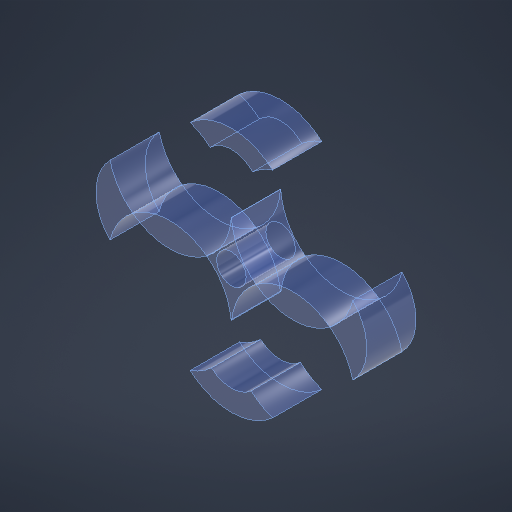
# Autodesk Inventor part: Peça2
Saved by Autodesk Inventor 2026.1 (Build 301233000, 233)
## iProperties
Created: 2025-10-22
Part Number: Peça2
Material: Água
Document SubType Name: Modeling
Designer: Pc
Density: 0.9983 g/cm^3
Appearance: Azul tropical
Author: Pc
Autodesk Inventor part; units mm, degrees
ref_plane "YZ Plane" through (0, 0, 0) normal (1, 0, 0) x (0, 1, 0)
ref_plane "XZ Plane" through (0, 0, 0) normal (0, 1, 0) x (-1, 0, 0)
ref_plane "XY Plane" through (0, 0, 0) normal (0, 0, 1) x (1, 0, 0)
sketch "Esboço1" plane through (0, 0, 0) normal (0, 0, 1) x (1, 0, 0)
  line L0 (30.3854, 49.745) -> (30.3854, 49.745)
  line L1 (42.8854, 37.245) -> (42.8854, 12.245)
  line L2 (30.3854, -0.255) -> (30.3854, -0.255)
  line L3 (17.8854, 12.245) -> (17.8854, 37.245)
  circle A0 centre (30.3854, 25) radius 3
  circle A1 centre (30.3854, 40) radius 6
  circle A2 centre (30.3854, 10) radius 6
  line L4 (47.8854, 34.745) -> (42.8854, 34.745)
  line L5 (42.8854, 34.745) -> (42.8854, 14.745)
  line L6 (42.8854, 14.745) -> (47.8854, 14.745)
  line L7 (57.8854, 24.745) -> (57.8854, 24.745)
  line L8 (12.8854, 34.745) -> (17.8854, 34.745)
  line L9 (17.8854, 34.745) -> (17.8854, 14.745)
  line L10 (17.8854, 14.745) -> (12.8854, 14.745)
  line L11 (2.8854, 24.745) -> (2.8854, 24.745)
  arc A3 (12.8854, 34.745) -> (2.8854, 24.745) centre (12.8854, 24.745) ccw
  arc A4 (2.8854, 24.745) -> (12.8854, 14.745) centre (12.8854, 24.745) ccw
  arc A5 (47.8854, 14.745) -> (57.8854, 24.745) centre (47.8854, 24.745) ccw
  arc A6 (57.8854, 24.745) -> (47.8854, 34.745) centre (47.8854, 24.745) ccw
  arc A7 (30.3854, 49.745) -> (17.8854, 37.245) centre (30.3854, 37.245) ccw
  arc A8 (42.8854, 37.245) -> (30.3854, 49.745) centre (30.3854, 37.245) ccw
  arc A9 (17.8854, 12.245) -> (30.3854, -0.255) centre (30.3854, 12.245) ccw
  arc A10 (30.3854, -0.255) -> (42.8854, 12.245) centre (30.3854, 12.245) ccw
  point P0 (0, 0)
  point P1 (17.8854, 49.745)
  point P2 (42.8854, -0.255)
  point P3 (42.8854, 49.745)
  point P4 (30.3854, 49.745)
  point P5 (30.3854, -0.255)
  point P6 (57.8854, 34.745)
  point P7 (57.8854, 14.745)
  point P8 (2.8854, 34.745)
  point P9 (2.8854, 14.745)
  point P10 (30.3854, -0.255)
  dimension "d0" = 50
  dimension "d1" = 25
  dimension "d2" = 6
  dimension "d3" = 12
  dimension "d4" = 12
  dimension "d8" = 20
  dimension "d9" = 15
  dimension "d11" = 15
  dimension "d12" = 20
  dimension "d13" = 10
  dimension "d14" = 12.5
  constraints: 24 end point, 18 point on line, 16 point on circle, 16 tangent, 11 centre point, 6 equal radius, 6 parallel, 3 horizontal, 3 perpendicular, 2 midpoint
  measures "d0" distance of point (42.885, 49.745) point (42.885, -0.255)
  measures "d1" distance of point (17.885, 49.745) point (42.885, 49.745)
  measures "d2" diameter of A0
  measures "d3" diameter of A1
  measures "d4" diameter of A2
  measures "d8" distance of point (57.885, 14.745) point (57.885, 34.745)
  measures "d9" distance of L5.end point (57.885, 14.745)
  measures "d11" distance of point (2.885, 34.745) L8.end
  measures "d12" distance of point (2.885, 14.745) point (2.885, 34.745)
  measures "d13" radius of A3
  measures "d14" radius of A7
extrude "Extrusão1" add sketch "Esboço1" along normal blind 10
sketch "Esboço2" plane through (0, 0, 10) normal (0, 0, 1) x (1, 0, 0)
  line L0 (17.8854, 34.745) -> (12.8854, 34.745) projected
  circle A0 centre (17.8854, 34.745) radius 12.5
  line L1 (47.8854, 34.745) -> (42.8854, 34.745) projected
  circle A1 centre (42.8854, 34.745) radius 12.5
  line L2 (42.8854, 12.245) -> (42.8854, 14.745) projected
  circle A2 centre (42.8854, 14.745) radius 12.5
  line L3 (17.8854, 14.745) -> (17.8854, 12.245) projected
  circle A3 centre (17.8854, 14.745) radius 12.5
  point P0 (0, 0)
  point P1 (10.3854, 24.745)
  point P2 (25.3854, 24.745)
  point P3 (30.3854, 34.745)
  point P4 (30.3854, 14.745)
  point P5 (35.3854, 24.745)
  point P6 (50.3854, 24.745)
  dimension "d17" = 25
  dimension "d18" = 25
  dimension "d19" = 25
  dimension "d20" = 25
  constraints: 4 centre point
  measures "d17" diameter of A0
  measures "d18" diameter of A1
  measures "d19" diameter of A2
  measures "d20" diameter of A3
extrude "Extrusão2" cut sketch "Esboço2" against normal blind 10 contours A0 A3 | A1 A2 | A0 A3 | A1 A2 picked at (18.0099, 40.5178) picked at (42.8854, 40.5176) picked at (18.0099, 8.9722) picked at (42.8854, 8.9724)
